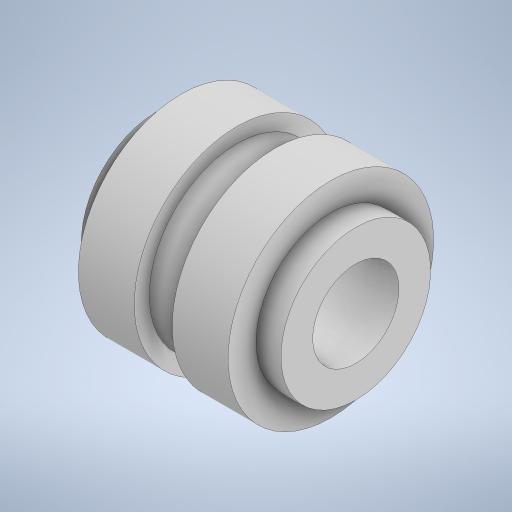
# Autodesk Inventor part: Pieza2-Tarea2
Saved by Autodesk Inventor 2024 (Build 280153000, 153)
## iProperties
Created: 2024-02-22
Part Number: Pieza2-Tarea2
Material: Genérico
Document SubType Name: Modeling
Designer: Diegolap
Density: 1 g/cm^3
Appearance: Valor por defecto
Author: Diegolap
Autodesk Inventor part; units mm, degrees
ref_plane "YZ Plane" through (0, 0, 0) normal (1, 0, 0) x (0, 1, 0)
ref_plane "XZ Plane" through (0, 0, 0) normal (0, 1, 0) x (-1, 0, 0)
ref_plane "XY Plane" through (0, 0, 0) normal (0, 0, 1) x (1, 0, 0)
sketch "Boceto1" plane through (0, 0, 0) normal (0, 0, 1) x (1, 0, 0)
  line L0 (0, 0) -> (6.35, 0)
  line L1 (6.35, 0) -> (6.35, 19.05)
  line L2 (6.35, 19.05) -> (0, 19.05)
  line L3 (0, 19.05) -> (0, 0)
  line L4 (6.35, 0) -> (20.574, 0)
  line L5 (20.574, 0) -> (20.574, 26.162)
  line L6 (20.574, 26.162) -> (6.35, 26.162)
  line L7 (6.35, 26.162) -> (6.35, 0)
  line L8 (20.574, 0) -> (30.226, 0)
  line L9 (30.226, 0) -> (30.226, 22.352)
  line L10 (30.226, 22.352) -> (20.574, 22.352)
  line L11 (20.574, 22.352) -> (20.574, 0)
  line L12 (30.226, 0) -> (44.45, 0)
  line L13 (44.45, 0) -> (44.45, 26.162)
  line L14 (44.45, 26.162) -> (30.226, 26.162)
  line L15 (30.226, 26.162) -> (30.226, 0)
  line L16 (44.45, 0) -> (50.8, 0)
  line L17 (50.8, 0) -> (50.8, 19.05)
  line L18 (50.8, 19.05) -> (44.45, 19.05)
  line L19 (44.45, 19.05) -> (44.45, 0)
  line L20 (0, 0) -> (50.8, 0)
  point P0 (30.226, 22.352)
  point P1 (6.35, 19.05)
  dimension "d2" = 19.05
  dimension "d3" = 26.162
  dimension "d4" = 9.652
  dimension "d5" = 50.8
  dimension "d6" = 14.224
  dimension "d7" = 6.35
  dimension "d8" = 3.81
  constraints: 42 end point, 10 parallel, 6 horizontal, 5 perpendicular, 2 point on line, 1 coincident, 1 collinear
  measures "d2" distance of L2.end L0.start
  measures "d3" distance of L6.end L0.end
  measures "d4" distance of L9.end L10.end
  measures "d5" distance of L2.end L17.end
  measures "d6" distance of L0.end L4.end
  measures "d7" distance of L0.start L0.end
  measures "d8" distance between parallel lines of L14 L10
revolve "Revolución1" add sketch "Boceto1" angle 360 about axis through (0, 0, 0) along (1, 0, 0)
sketch "Boceto2" plane through (0, 0, 0) normal (-1, 0, 0) x (0, 0, 1)
  circle A0 centre (0, 0) radius 10.9883
  constraints: 1 centre point, 1 coincident
extrude "Extrusión1" cut sketch "Boceto2" against normal blind 50.8
equation "\"d2\" = 0.5 * DistC"
equation "\"d3\" = 0.5 * DistA"
equation "\"d4\" = DistE"
equation "\"d5\" = DistB"
equation "\"d6\" = DistX"
equation "\"d7\" = DistD - DistX"
equation "\"d10\" = DistB"
equation "\"DistA\" = 52.324"
equation "\"DistB\" = 50.8"
equation "\"DistC\" = 38.1"
equation "\"DistD\" = 20.574"
equation "\"DistE\" = 9.652"
equation "\"DistX\" = 14.224"
